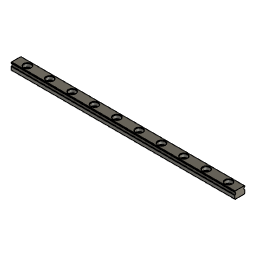
mgn9c rail 200mm (Autodesk Fusion 360 design; units mm, degrees)
Autodesk Fusion 360 part; units mm, degrees
note: some values were not read from the file. Set by a fixed rule: which face or edge a step refers to.
sketch "Sketch1" plane through (0, 0, 0) normal (1, 0, 0) x (0, 1, 0)
  line L0 (0, 0) -> (9, 0)
  line L1 (9, 0) -> (9, 6.5)
  line L2 (9, 6.5) -> (0, 6.5)
  line L3 (0, 6.5) -> (0, 0)
  circle A0 centre (9, 4.468) radius 0.9525
  circle A1 centre (0, 4.468) radius 0.9525
  dimension "d1" = 9
  dimension "d2" = 6.5
  dimension "d3" = 1.905
  dimension "d4" = 1.905
  dimension "d5" = 2.032
  dimension "d6" = 2.032
  constraint horizontal L0
  constraint vertical L1
  constraint horizontal L2
  constraint vertical L3
  constraint coincident L0.start L3.end
  constraint coincident L1 A0.centre
  constraint coincident L3 A1.centre
  measures "d1" distance of L0.start L0.end
  measures "d2" distance of L0.end L1.end
  measures "d3" diameter of A0
  measures "d4" diameter of A1
  measures "d5" distance of L2.end A1.centre
  measures "d6" distance of L1.end A0.centre
extrude "Extrude1" add sketch "Sketch1" along normal blind 200 contours L0 L1 L2 L3 A0 A1
fillet "Fillet1" radius 0.381 4 edges at (100, 9, 6.5) (100, 9, 0) (100, 0, 6.5) (100, 0, 0)
fillet "Fillet1" radius 0.381 4 edges at (100, 9, 3.5155) (100, 9, 5.4205) (100, 0, 3.5155) (100, 0, 5.4205)
sketch "Sketch2" plane through (0, 0, 6.5) normal (0, 0, 1) x (-1, 0, 0)
  line L0 (0, -0.381) -> (-200, -0.381)
  line L1 (-200, -0.381) -> (-200, -8.619)
  line L2 (-200, -8.619) -> (0, -8.619)
  line L3 (0, -8.619) -> (0, -0.381)
  line L4 (0, -4.5) -> (-200, -4.5)
  circle A0 centre (-10, -4.5) radius 3
  dimension "d13" = 6
  dimension "d22" = 10
  constraint midpoint L3 L4.start
  constraint midpoint L1 L4.end
  constraint coincident L4 A0.centre
  measures "d13" diameter of A0
  measures "d22" distance of L4.start A0.centre
extrude "Extrude2" cut sketch "Sketch2" against normal blind 3.5 contours L4 A0 | L4 A0
sketch "Sketch3" plane through (0, 0, 3) normal (0, 0, 1) x (-1, 0, 0)
  circle A0 centre (-10, -4.5) radius 3
  circle A1 centre (-10, -4.5) radius 1.75
  dimension "d16" = 3.5
  constraint concentric A0 A1
  measures "d16" diameter of A1
extrude "Extrude3" cut sketch "Sketch3" against normal blind 15.24 contours A1
pattern_path "PathPattern1" count 10 spacing 20 from (0, 8.619, 6.5) along 1 edges at (100, 8.619, 6.5) of "Extrude2", "Extrude3"
chamfer "Chamfer1" distance 0.381 angle 45 3 edges at (11.6316, 5.1328, 0) (31.6316, 5.1328, 0) (51.6316, 5.1328, 0) 3 faces at (7.0037, 4.3505, 5.3333) (27.0037, 4.3505, 5.3333) (47.0037, 4.3505, 5.3333)
chamfer "Chamfer2" distance 0.381 angle 45 4 edges at (71.6316, 5.1328, 0) (91.6316, 5.1328, 0) (111.6316, 5.1328, 0) (131.6316, 5.1328, 0) 4 faces at (71.2339, 1.7655, 4.1667) (91.2339, 1.7655, 4.1667) (111.2339, 1.7655, 4.1667) (130.9555, 7.3438, 4.1667)
chamfer "Chamfer3" distance 0.381 angle 45 3 edges at (191.6316, 5.1328, 0) (171.6316, 5.1328, 0) (151.6316, 5.1328, 0) 3 faces at (150.9555, 7.3438, 4.1667) (170.9555, 7.3438, 4.1667) (190.9555, 7.3438, 4.1667)
